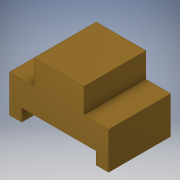
# Autodesk Inventor part: Brass Object
Saved by Autodesk Inventor 2017 (Build 210142000, 142)
## iProperties
Created: 2020-03-10
Part Number: Brass Object
Material: Brass, Soft Yellow
Document SubType Name: Modeling
Designer: 10042265
Density: 8.47 g/cm^3
Appearance: Brass - Satin
Author: 10042265
Autodesk Inventor part; units mm, degrees
ref_plane "YZ Plane" through (0, 0, 0) normal (1, 0, 0) x (0, 1, 0)
ref_plane "XZ Plane" through (0, 0, 0) normal (0, 1, 0) x (-1, 0, 0)
ref_plane "XY Plane" through (0, 0, 0) normal (0, 0, 1) x (1, 0, 0)
sketch "Sketch1" plane through (0, 0, 0) normal (0, 0, 1) x (1, 0, 0)
  line L0 (0, 0) -> (6.35, 0)
  line L1 (6.35, 0) -> (6.35, 6.35)
  line L2 (6.35, 6.35) -> (44.45, 6.35)
  line L3 (44.45, 6.35) -> (44.45, 0)
  line L4 (44.45, 0) -> (50.8, 0)
  line L5 (50.8, 0) -> (50.8, 19.05)
  line L6 (50.8, 19.05) -> (38.1, 19.05)
  line L7 (38.1, 19.05) -> (38.1, 31.75)
  line L8 (38.1, 31.75) -> (12.7, 31.75)
  line L9 (12.7, 31.75) -> (12.7, 19.05)
  line L10 (12.7, 19.05) -> (0, 19.05)
  line L11 (0, 19.05) -> (0, 0)
  dimension "d1" = 6.35
  dimension "d2" = 6.35
  dimension "d3" = 38.1
  dimension "d4" = 6.35
  dimension "d5" = 19.05
  dimension "d6" = 12.7
  dimension "d7" = 12.7
  dimension "d8" = 25.4
  constraints: 24 end point, 9 perpendicular, 3 point on line, 2 horizontal
  measures "d1" distance of L0.start L0.end
  measures "d2" distance of L0.end L1.end
  measures "d3" distance of L1.end L2.end
  measures "d4" distance of L3.end L4.end
  measures "d5" distance of L4.end L5.end
  measures "d6" distance of L5.end L6.end
  measures "d7" distance of L6.end L7.end
  measures "d8" distance of L7.end L8.end
extrude "Extrusion1" add sketch "Sketch1" along normal blind 31.75
body "Solid1"
